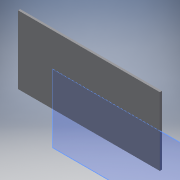
# Autodesk Inventor part: top2b
Saved by Autodesk Inventor 2017 (Build 210142000, 142)
## iProperties
Created: 2016-12-08
Part Number: top2b
Material: Generic
Document SubType Name: Modeling
Designer: SDL
Density: 1 g/cm^3
Appearance: Default
Author: SDL
Autodesk Inventor part; units mm, degrees
ref_plane "YZ Plane" through (0, 0, 0) normal (1, 0, 0) x (0, 1, 0)
ref_plane "XZ Plane" through (0, 0, 0) normal (0, 1, 0) x (-1, 0, 0)
ref_plane "XY Plane" through (0, 0, 0) normal (0, 0, 1) x (1, 0, 0)
sketch "Sketch1" plane through (0, 0, 0) normal (0, 0, 1) x (1, 0, 0)
  line L0 (0, 0) -> (133, 0)
  line L1 (133, 0) -> (133, 64)
  line L2 (133, 64) -> (0, 64)
  line L3 (0, 64) -> (0, 0)
  line L4 (0, 64) -> (0, 62.5)
  line L5 (81.5, 62.5) -> (51.5, 62.5)
  line L6 (51.5, 62.5) -> (51.5, 59.5)
  line L7 (51.5, 59.5) -> (81.5, 59.5)
  line L8 (81.5, 59.5) -> (81.5, 62.5)
  dimension "d0" = 133
  dimension "d1" = 64
  dimension "d6" = 30
  dimension "d7" = 3
  constraints: 18 end point, 4 parallel, 2 horizontal, 2 perpendicular, 1 point on line
  measures "d0" distance of L2.end L1.end
  measures "d1" distance of L1.end L0.end
  measures "d6" distance of L7.end L6.end
  measures "d7" distance of L6.end L5.end
extrude "Extrusion1" add sketch "Sketch1" along normal blind 2 contours L3 L2 L1 L0 | L8 L7 L6 L5
sketch "Sketch2" plane through (0, 0, 2) normal (0, 0, 1) x (1, 0, 0)
  line L0 (133, 64) -> (0, 64) projected
  line L1 (0, 64) -> (0, 0) projected
  line L2 (81.5, 62.5) -> (51.5, 62.5)
  line L3 (51.5, 62.5) -> (51.5, 59)
  line L4 (51.5, 59) -> (81.5, 59)
  line L5 (81.5, 59) -> (81.5, 62.5)
  dimension "d12" = 30
  dimension "d13" = 3.5
  constraints: 8 end point, 2 parallel, 1 horizontal, 1 perpendicular
  measures "d12" distance of L4.end L3.end
  measures "d13" distance of L3.end L2.end
extrude "Extrusion2" add sketch "Sketch2" against normal blind 3
body "Solid1"
